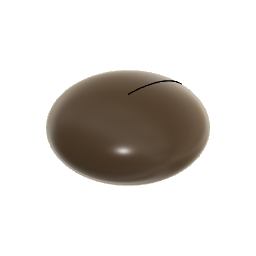
brown_M&M (Autodesk Fusion 360 design; units mm, degrees)
Autodesk Fusion 360 part; units mm, degrees
note: some values were not read from the file. Set by a fixed rule: which sketch regions a step uses.
sketch "Smartie Outline" plane through (0, 0, 0) normal (1, 0, 0) x (0, 1, 0)
  spline S0 degree 5 poles (-7, 0) (-7, 0.2185) (-6.9298, 0.6556) (-6.6141, 1.3008) (-5.7894, 2.0984) (-4.1968, 2.8947) (-2.2027, 3.4101) (0, 3.5892) (2.2027, 3.4101) (4.1968, 2.8947) (5.7894, 2.0984) (6.8202, 1.1014) (7.1783, 0) (6.8202, -1.1014) (5.7894, -2.0984) (4.1968, -2.8947) (2.2027, -3.4101) (0, -3.5892) (-2.2027, -3.4101) (-4.1968, -2.8947) (-5.7894, -2.0984) (-6.6141, -1.3008) (-6.9298, -0.6556) (-7, -0.2185) (-7, 0) knots 0 0 0 0 0 0 0.05 0.1 0.15 0.2 0.25 0.3 0.35 0.4 0.45 0.5 0.55 0.6 0.65 0.7 0.75 0.8 0.85 0.9 0.95 1 1 1 1 1 1
  line L0 (0, -3.5) -> (0, 3.5)
  point P0 (0, 3.5)
  point P1 (7, 0)
  point P2 (0, -3.5)
  dimension "d3" = 3.5
  dimension "d4" = 3.5
  dimension "d5" = 7
  dimension "d6" = 7
  constraint coincident P2 L0.start
  constraint coincident P0 L0.end
  constraint vertical L0
  measures "d3" distance of origin L0.end
  measures "d4" distance of origin P2
  measures "d5" distance of origin S0.start
  measures "d6" distance of origin P1
revolve "Revolve1" add sketch "Smartie Outline" angle 360 about axis through (0, 0, -3.5) along (0, 0, 1) contours S0 L0 picked at (-0.9633, -1.1535)
equation "mmWidth = 14 mm" comment "Major axis of the M&M"
equation "mmHeight = 7 mm" comment "Minor axis of the M&M"
equation "d3 = mmHeight / 2"
equation "d4 = mmHeight / 2"
equation "d5 = mmWidth / 2"
equation "d6 = mmWidth / 2"
named bodies: "Brown M&M"
